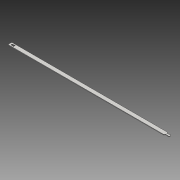
# Autodesk Inventor part: Пластина LED(New6)-развёртка
Saved by Autodesk Inventor 2016 (Build 200138000, 138)
## iProperties
Created: 2020-03-10
Part Number: Пластина LED(New6)-развёртка
Material: Типовые
Document SubType Name: Modeling
Designer: Рябов
Density: 1 g/cm^3
Appearance: По умолчанию
Mass: 11.1589 g
Surface Area: 130.667 cm^2
Volume: 11.1589 cm^3
Author: Рябов
Autodesk Inventor part; units mm, degrees
ref_plane "YZ Plane" through (0, 0, 0) normal (1, 0, 0) x (0, 1, 0)
ref_plane "XZ Plane" through (0, 0, 0) normal (0, 1, 0) x (-1, 0, 0)
ref_plane "XY Plane" through (0, 0, 0) normal (0, 0, 1) x (1, 0, 0)
sketch "Эскиз1" plane through (0, 0, 0) normal (0, 0, 1) x (1, 0, 0)
  line L0 (-251.3272, 12) -> (251.3272, 12)
  line L1 (251.3272, 12) -> (251.3272, 0)
  line L2 (251.3272, 0) -> (-251.3272, 0)
  line L3 (-251.3272, 0) -> (-251.3272, 12)
  point P0 (0, 0)
  point P1 (0, 0)
  dimension "d0" = 12
  dimension "d1" = 502.6544
  constraints: 8 end point, 2 parallel, 1 coincident, 1 horizontal, 1 midpoint, 1 perpendicular
  measures "d0" distance of L0.end L1.end
  measures "d1" distance of L0.start L0.end
extrude "Выдавливание1" add sketch "Эскиз1" against normal blind 2
sketch "Эскиз4" plane through (0, 0, 0) normal (0, 0, 1) x (1, 0, 0)
  arc A0 (-243.8272, 8.5) -> (-243.8272, 3.5) centre (-243.8272, 6) ccw projected
  line L0 (-243.8272, 8.5) -> (-239.948, 8.5) projected
  arc A1 (-239.948, 8.5) -> (-239.1165, 8.9444) centre (-239.948, 9.5) ccw projected
  arc A2 (-236.8272, 8.25) -> (-239.1165, 8.9444) centre (-238.0772, 8.25) ccw projected
  line L1 (-236.8272, 8.25) -> (-236.8272, 3.75) projected
  arc A3 (-239.1165, 3.0556) -> (-236.8272, 3.75) centre (-238.0772, 3.75) ccw projected
  arc A4 (-239.1165, 3.0556) -> (-239.948, 3.5) centre (-239.948, 2.5) ccw projected
  line L2 (-239.948, 3.5) -> (-243.8272, 3.5) projected
  arc A5 (217.9113, 0) -> (219.9113, 2) centre (217.9113, 2) ccw construction
  line L3 (219.9113, 2.25) -> (219.9113, 2) construction
  arc A6 (221.1613, 3.5) -> (219.9113, 2.25) centre (221.1613, 2.25) ccw construction
  line L4 (227.4618, 3.5) -> (221.1613, 3.5) construction
  arc A7 (227.4618, 3.5) -> (227.4618, 8.5) centre (229.9113, 6) ccw construction
  line L5 (221.1613, 8.5) -> (227.4618, 8.5) construction
  arc A8 (219.9113, 9.75) -> (221.1613, 8.5) centre (221.1613, 9.75) ccw construction
  line L6 (219.9113, 10) -> (219.9113, 9.75) construction
  arc A9 (219.9113, 10) -> (217.9113, 12) centre (217.9113, 10) ccw construction
  line L7 (-249.3272, 12) -> (217.9113, 12) construction
  arc A10 (-249.3272, 12) -> (-251.3272, 10) centre (-249.3272, 10) ccw construction
  line L8 (-251.3272, 2) -> (-251.3272, 10) construction
  arc A11 (-251.3272, 2) -> (-249.3272, 0) centre (-249.3272, 2) ccw construction
  line L9 (217.9113, 0) -> (-249.3272, 0) construction
  line L10 (252.5772, 8.5) -> (258.8777, 8.5) projected
  arc A12 (258.8777, 3.5) -> (258.8777, 8.5) centre (261.3272, 6) ccw projected
  line L11 (258.8777, 3.5) -> (252.5772, 3.5) projected
  arc A13 (252.5772, 3.5) -> (251.3272, 2.25) centre (252.5772, 2.25) ccw projected
  arc A14 (251.3272, 9.75) -> (252.5772, 8.5) centre (252.5772, 9.75) ccw projected
  line L12 (251.3272, 9.75) -> (251.3272, 2.25)
  line L13 (251.3272, 12) -> (251.3272, 0) construction
  point P0 (0, 0)
  constraints: 2 end point, 1 collinear
extrude "Выдавливание4" add sketch "Эскиз4" against normal up to surface (2 mm away) contours L10 A12 L11 A13 L12 A14
extrude "Выдавливание5" cut sketch "Эскиз4" against normal blind 10 contours L0 A1 A2 L1 A3 A4 L2 A0
fillet "Сопряжение2" radius 2 4 edges at (251.3272, 0, -1) (251.3272, 12, -1) (-251.3272, 0, -1) (-251.3272, 12, -1)
sketch "Эскиз2" plane through (0, 0, 0) normal (0, 0, 1) x (1, 0, 0)
  line L0 (-251.3272, 12) -> (251.3272, 12) projected
  line L1 (-251.3272, 0) -> (-251.3272, 12) projected
  line L2 (251.3272, 0) -> (-251.3272, 0) projected
  line L3 (251.3272, 12) -> (251.3272, 0) projected
  line L4 (0, 0) -> (0, 12)
  constraints: 2 end point, 1 midpoint
